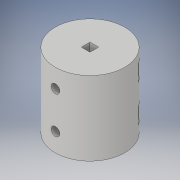
# Autodesk Inventor part: Coupler 5x8
Saved by Autodesk Inventor 2019 (Build 230136000, 136)
## iProperties
Created: 2020-02-08
Part Number: Coupler 5x8
Material: Genérico
Document SubType Name: Modeling
Designer: Diego Guillén
Density: 1 g/cm^3
Appearance: Valor por defecto
Author: Diego Guillén
Autodesk Inventor part; units mm, degrees
ref_plane "YZ Plane" through (0, 0, 0) normal (1, 0, 0) x (0, 1, 0)
ref_plane "XZ Plane" through (0, 0, 0) normal (0, 1, 0) x (-1, 0, 0)
ref_plane "XY Plane" through (0, 0, 0) normal (0, 0, 1) x (1, 0, 0)
sketch "Boceto1" plane through (0, 0, 0) normal (0, 1, 0) x (-1, 0, 0)
  circle A0 centre (0, 0) radius 12
  dimension "d0" = 24
  constraints: 1 centre point, 1 coincident
  measures "d0" diameter of A0
extrude "Extrusión1" add sketch "Boceto1" along normal blind 25.6
sketch "Boceto2" plane through (0, 25.6, 0) normal (0, 1, 0) x (1, 0, 0)
  point P0 (0, 0)
  point P1 (0, 0)
  constraints: 1 coincident
hole "Agujero1" at (0, 25.6, 0) direction (0, -1, 0) diameter 5 depth 35 tip angle 118
sketch "Boceto3" plane through (0, 25.6, 0) normal (0, 1, 0) x (1, 0, 0)
  point P0 (0, 0)
  point P1 (0, 0)
  constraints: 1 coincident
hole "Agujero2" at (0, 25.6, 0) direction (0, -1, 0) diameter 8 depth 12.8
sketch "Boceto4" plane through (0, 0, 0) normal (1, 0, 0) x (0, 1, 0)
  line L0 (9.2, -7) -> (3.6, -7)
  line L1 (3.6, -7) -> (3.6, -9.42)
  line L2 (3.6, -9.42) -> (9.2, -9.42)
  line L3 (9.2, -9.42) -> (9.2, -7)
  line L4 (25.6, -12) -> (25.6, 12) construction
  line L5 (0, 12) -> (0, -12) construction
  line L6 (12.8, -2.5) -> (12.8, 2.5) construction
  line L7 (0, -2.5) -> (0, 2.5) construction
  line L8 (19.2, 26.4321) -> (19.2, -18.0419) construction
  line L9 (6.4, 12.9466) -> (6.4, -18.0419) construction
  line L10 (22, -7) -> (16.4, -7)
  line L11 (16.4, -7) -> (16.4, -9.42)
  line L12 (16.4, -9.42) -> (22, -9.42)
  line L13 (22, -9.42) -> (22, -7)
  line L14 (0, -2.5) -> (0, 2.5) construction
  point P0 (0, 0)
  point P1 (6.4, -7)
  point P2 (19.2, -7)
  dimension "d17" = 5.6
  dimension "d18" = 2.42
  dimension "d19" = 6.4
  dimension "d20" = 6.4
  dimension "d21" = 5.6
  dimension "d22" = 2.42
  dimension "d23" = 9.42
  dimension "d24" = 9.42
  constraints: 20 end point, 4 parallel, 2 horizontal, 2 midpoint, 2 perpendicular, 2 point on line, 2 vertical
  measures "d17" distance of L1.end L2.end
  measures "d18" distance of L0.end L1.end
  measures "d19" distance between parallel lines of L4 L8
  measures "d20" distance between parallel lines of L9 L5
  measures "d21" distance of L11.end L12.end
  measures "d22" distance of L10.end L11.end
  measures "d23" distance from line of L12 point (0, 0)
  measures "d24" distance from line of point (0, 0) L2
extrude "Extrusión2" cut sketch "Boceto4" along normal blind 10 and the other way blind 3
sketch "Boceto5" plane through (9.7468, 16.4, -7) normal (0, 0, -1) x (-1, 0, 0)
  line L0 (0, -7.2) -> (2.3128, -7.2) construction
  line L1 (2.3128, -7.2) -> (2.3128, -12.8) construction
  line L2 (2.3128, -12.8) -> (0, -12.8) construction
  line L3 (0, -12.8) -> (0, -7.2) construction
  line L4 (0, 5.6) -> (2.3128, 5.6) construction
  line L5 (2.3128, 5.6) -> (2.3128, 0) construction
  line L6 (2.3128, 0) -> (0, 0) construction
  line L7 (0, 0) -> (0, 5.6) construction
  line L8 (21.7468, 9.2) -> (-2.2532, 9.2) construction
  line L9 (-2.2532, -16.4) -> (21.7468, -16.4) construction
  point P0 (9.7468, -16.4)
  point P1 (9.7468, 2.8)
  point P2 (9.7468, -10)
  point P3 (2.3128, -10)
  point P4 (2.3128, 2.8)
  constraints: 2 horizontal alignment, 2 midpoint, 2 vertical alignment
hole "Agujero3" at (0, 19.2, -7) at (0, 6.4, -7) direction (0, 0, 1) diameter 3 end through all both
sketch "Boceto6" plane through (0, 12.8, 0) normal (0, 1, 0) x (1, 0, 0)
  circle A0 centre (0, 0) radius 4 construction
  circle A1 centre (0, 0) radius 12 construction
  circle A2 centre (0, 0) radius 2.5 construction
  line L0 (1.5, -1.5) -> (-1.5, -1.5)
  line L1 (-1.5, -1.5) -> (-1.5, 1.5)
  line L2 (-1.5, 1.5) -> (1.5, 1.5)
  line L3 (1.5, 1.5) -> (1.5, -1.5)
  line L4 (-1.5, 1.5) -> (1.5, -1.5) construction
  line L5 (1.5, 1.5) -> (-1.5, -1.5) construction
  circle A3 centre (0, 0) radius 4
  dimension "d36" = 3
  dimension "d37" = 3
  dimension "d38" = 8
  constraints: 12 end point, 2 coincident, 2 parallel, 1 centre point, 1 horizontal, 1 midpoint, 1 perpendicular
  measures "d36" distance of L2.end L0.start
  measures "d37" distance of L1.end L2.end
  measures "d38" diameter of A3
extrude "Extrusión3" add sketch "Boceto6" along normal up to surface (12.8 mm away)
equation "\"d20\" = d19"
equation "\"d24\" = d23"
